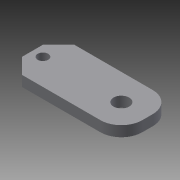
# Autodesk Inventor part: servo arm
Saved by Autodesk Inventor 2013 (Build 170138000, 138)
## iProperties
Created: 2017-01-26
Part Number: servo arm
Material: Generic
Document SubType Name: Modeling
Designer: Herman de Vries
Density: 1 g/cm^3
Author: Herman de Vries
Autodesk Inventor part; units mm, degrees
ref_plane "YZ Plane" through (0, 0, 0) normal (1, 0, 0) x (0, 1, 0)
ref_plane "XZ Plane" through (0, 0, 0) normal (0, 1, 0) x (-1, 0, 0)
ref_plane "XY Plane" through (0, 0, 0) normal (0, 0, 1) x (1, 0, 0)
sketch "Sketch1" plane through (0, 0, 0) normal (0, 0, 1) x (1, 0, 0)
  line L0 (0, 0) -> (22, 0)
  line L1 (22, 0) -> (22, 10)
  line L2 (22, 10) -> (0, 10)
  line L3 (0, 10) -> (0, 0)
  circle A0 centre (17, 5) radius 1.5
  circle A1 centre (2, 5) radius 1
  point P0 (22, 5)
  dimension "d0" = 22
  dimension "d1" = 10
  dimension "d2" = 3
  dimension "d3" = 2
  dimension "d4" = 15
  dimension "d5" = 5
  constraints: 8 end point, 2 centre point, 2 horizontal alignment, 2 parallel, 1 horizontal, 1 midpoint, 1 perpendicular
  measures "d0" distance of L2.end L1.end
  measures "d1" distance of L1.end L0.end
  measures "d2" diameter of A0
  measures "d3" diameter of A1
  measures "d4" distance of A0.centre A1.centre
  measures "d5" distance from line of L1 A0.centre
extrude "Extrusion1" add sketch "Sketch1" along normal blind 2
fillet "Fillet1" radius 4 2 edges at (22, 10, 1) (22, 0, 1)
chamfer "Chamfer1" distance 3 angle 45 2 edges at (0, 10, 1) (0, 0, 1)
body "Solid1"
